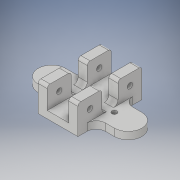
# Autodesk Inventor part: TestBracket
Saved by Autodesk Inventor 2018 (Build 220112000, 112)
## iProperties
Created: 2019-10-18
Part Number: TestBracket
Material: Generic
Document SubType Name: Modeling
Designer: anirudh
Density: 1 g/cm^3
Appearance: Default
Author: anirudh
Autodesk Inventor part; units mm, degrees
ref_plane "YZ Plane" through (0, 0, 0) normal (1, 0, 0) x (0, 1, 0)
ref_plane "XZ Plane" through (0, 0, 0) normal (0, 1, 0) x (-1, 0, 0)
ref_plane "XY Plane" through (0, 0, 0) normal (0, 0, 1) x (1, 0, 0)
sketch "Sketch1" plane through (0, 0, 0) normal (0, 1, 0) x (-1, 0, 0)
  circle A0 centre (-105.9111, 9.525) radius 1.75
  circle A1 centre (-71.9005, 9.525) radius 1.75
  circle A2 centre (-105.9111, 9.525) radius 1.75
  circle A3 centre (-71.9005, 9.525) radius 1.75
  line L0 (-62.3755, 0) -> (-115.4361, 0)
  line L1 (-62.3755, 19.05) -> (-115.4361, 19.05)
  arc A4 (-115.4361, 19.05) -> (-115.4361, 0) centre (-115.4361, 9.525) ccw
  arc A5 (-62.3755, 0) -> (-62.3755, 19.05) centre (-62.3755, 9.525) ccw
  point P0 (0, 0)
  constraints: 6 centre point, 4 end point, 4 point on circle, 2 concentric, 1 coincident
extrude "Extrusion1" add sketch "Sketch1" along normal blind 5.08
sketch "Sketch2" plane through (0, 5.08, 0) normal (0, 1, 0) x (1, 0, 0)
  line L0 (96.4058, -19.05) -> (96.4058, 0)
  line L1 (81.4058, 0) -> (81.4058, -19.05)
  line L2 (81.4058, 0) -> (81.4058, 12.7)
  line L3 (81.4058, 12.7) -> (96.4058, 12.7)
  line L4 (96.4058, 12.7) -> (96.4058, 0)
  line L5 (96.4058, -19.05) -> (96.4058, -31.75)
  line L6 (96.4058, -31.75) -> (81.4058, -31.75)
  line L7 (81.4058, -31.75) -> (81.4058, -19.05)
  line L8 (81.4058, 12.7) -> (81.4058, -31.75)
  line L9 (81.4058, -31.75) -> (96.4058, -31.75)
  line L10 (96.4058, -31.75) -> (96.4058, 12.7)
  line L11 (96.4058, 12.7) -> (81.4058, 12.7)
  point P0 (0, 0)
  point P1 (62.3755, -19.05)
  point P2 (115.4361, -19.05)
  dimension "d4" = 12.7
  dimension "d5" = 12.7
  constraints: 24 end point, 5 equal length, 2 point on line, 1 perpendicular, 1 vertical
  measures "d4" distance of L2.start L2.end
  measures "d5" distance of L5.start L5.end
extrude "Extrusion2" add sketch "Sketch2" against normal blind 5.08
sketch "Sketch3" plane through (0, 0, 0) normal (0, -1, 0) x (1, 0, 0)
  line L0 (81.4058, 19.05) -> (81.4058, 31.75) projected
  line L1 (81.4058, 31.75) -> (75.0558, 31.75)
  line L2 (75.0558, 31.75) -> (75.0558, -12.7)
  line L3 (75.0558, -12.7) -> (81.4058, -12.7)
  line L4 (81.4058, -12.7) -> (81.4058, 31.75)
  line L5 (81.4058, 31.75) -> (96.4058, 31.75) projected
  line L6 (96.4058, 31.75) -> (102.7558, 31.75)
  line L7 (102.7558, 31.75) -> (102.7558, -12.7)
  line L8 (102.7558, -12.7) -> (96.4058, -12.7)
  line L9 (96.4058, -12.7) -> (96.4058, 31.75)
  point P0 (0, 0)
  dimension "d8" = 6.35
  dimension "d9" = 6.35
  constraints: 16 end point, 4 parallel, 2 horizontal, 2 perpendicular, 1 point on line
  measures "d8" distance of L3.end L2.end
  measures "d9" distance of L7.end L8.end
extrude "Extrusion3" add sketch "Sketch3" against normal blind 20.08
sketch "Sketch4" plane through (0, 20.08, 0) normal (0, 1, 0) x (1, 0, 0)
  line L0 (75.0558, -31.75) -> (75.0558, -19.05) projected
  line L1 (75.0558, -15.1567) -> (102.7558, -15.1567)
  line L2 (102.7558, -31.75) -> (102.7558, 12.7) projected
  line L3 (75.0558, 0) -> (75.0558, 12.7) projected
  line L4 (75.0558, -3.8875) -> (102.7558, -3.8875)
  line L5 (102.7558, -3.8875) -> (102.7558, -15.1567)
  line L6 (102.7558, -15.1567) -> (75.0558, -15.1567)
  line L7 (75.0558, -15.1567) -> (75.0558, -3.8875)
  point P0 (0, 0)
  constraints: 10 end point, 2 parallel, 1 horizontal, 1 perpendicular, 1 point on line
extrude "Extrusion4" cut sketch "Sketch4" against normal blind 15
fillet "Fillet1" radius 3.175 4 edges at (99.5808, 5.08, 15.1567) (78.2308, 5.08, 15.1567) (78.2308, 5.08, 3.8875) (99.5808, 5.08, 3.8875)
fillet "Fillet2" radius 6.35 4 edges at (102.7558, 2.54, 19.05) (102.7558, 2.54, 0) (75.0558, 2.54, 0) (75.0558, 2.54, 19.05)
sketch "Sketch5" plane through (75.0558, 0, -12.7) normal (-1, 0, 0) x (0, 0, 1)
  line L0 (0, 5.08) -> (19.7625, 5.08) projected
  line L1 (0, 0) -> (0, 20.08) projected
  line L2 (27.8567, 8.255) -> (27.8567, 20.08) projected
  line L3 (44.45, 5.08) -> (24.6817, 5.08) projected
  circle A0 centre (8.2937, 12.58) radius 1.85
  circle A1 centre (36.1533, 12.58) radius 1.85
  point P0 (12.7, 0)
  point P1 (16.5875, 20.08)
  dimension "d16" = 3.7
  dimension "d17" = 3.7
  constraints: 2 centre point
  measures "d16" diameter of A0
  measures "d17" diameter of A1
extrude "Extrusion5" cut sketch "Sketch5" against normal blind 37.225
fillet "Fillet3" radius 1.905 8 edges at (99.5808, 20.08, -12.7) (99.5808, 20.08, 3.8875) (99.5808, 20.08, 15.1567) (99.5808, 20.08, 31.75) (78.2308, 20.08, 31.75) (78.2308, 20.08, 15.1567) (78.2308, 20.08, 3.8875) (78.2308, 20.08, -12.7)
body "Solid1"
